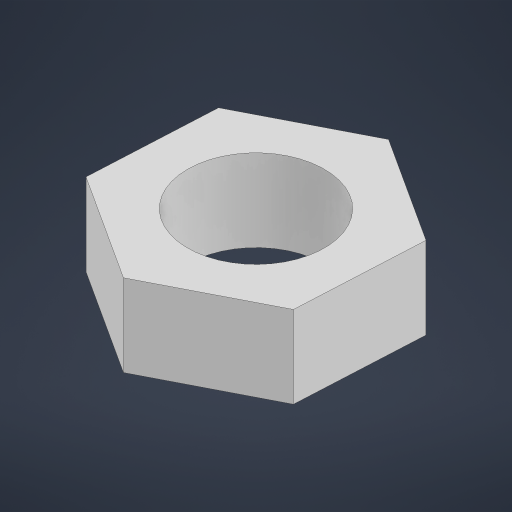
# Autodesk Inventor part: oc5mm
Saved by Autodesk Inventor 2023 (Build 270158000, 158)
## iProperties
Created: 2023-09-13
Part Number: oc5mm
Material: Generic
Document SubType Name: Modeling
Designer: philo
Density: 1 g/cm^3
Appearance: Default
Author: philo
Autodesk Inventor part; units mm, degrees
ref_plane "YZ Plane" through (0, 0, 0) normal (1, 0, 0) x (0, 1, 0)
ref_plane "XZ Plane" through (0, 0, 0) normal (0, 1, 0) x (-1, 0, 0)
ref_plane "XY Plane" through (0, 0, 0) normal (0, 0, 1) x (1, 0, 0)
sketch "Sketch1" plane through (0, 0, 0) normal (0, 1, 0) x (-1, 0, 0)
  circle A0 centre (0, 0) radius 2.5
  line L0 (3.8781, -2.5087) -> (-0.2335, -4.6129)
  line L1 (-0.2335, -4.6129) -> (-4.1117, -2.1042)
  line L2 (-4.1117, -2.1042) -> (-3.8781, 2.5087)
  line L3 (-3.8781, 2.5087) -> (0.2335, 4.6129)
  line L4 (0.2335, 4.6129) -> (4.1117, 2.1042)
  line L5 (4.1117, 2.1042) -> (3.8781, -2.5087)
  dimension "d0" = 5
  dimension "d1" = 4
  constraints: 12 end point, 2 coincident, 1 centre point, 13 other
  measures "d0" diameter of A0
  measures "d1" distance from line of point (0, 0) L5
extrude "Extrusion1" add sketch "Sketch1" along normal blind 3
body "Solid1"
